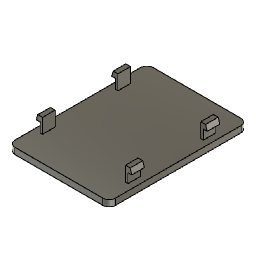
Bottom (Autodesk Fusion 360 design; units mm, degrees)
Autodesk Fusion 360 part; units mm, degrees
sketch "Sketch1" plane through (0, 0, 0) normal (0, 0, 1) x (1, 0, 0)
  line L0 (0, 0) -> (80, 0)
  line L1 (80, 0) -> (80, 110)
  line L2 (80, 110) -> (0, 110)
  line L3 (0, 110) -> (0, 0)
  dimension "d1" = 80
  dimension "d2" = 110
  constraint horizontal L0
  constraint vertical L1
  constraint horizontal L2
  constraint vertical L3
  constraint coincident L0.start L3.end
  measures "d1" distance of L0.start L0.end
  measures "d2" distance of L0.start L2.end
extrude "Extrude1" add sketch "Sketch1" along normal blind 5
fillet "Fillet1" radius 5 4 edges at (80, 0, 2.5) (0, 0, 2.5) (80, 110, 2.5) (0, 110, 2.5)
sketch "Sketch2" plane through (0, 0, 5) normal (0, 0, 1) x (-1, 0, 0)
  arc A0 (-5, -110) -> (0, -105) centre (-5, -105) ccw
  line L0 (0, -105) -> (0, -5)
  arc A1 (0, -5) -> (-5, 0) centre (-5, -5) ccw
  line L1 (-5, 0) -> (-75, 0)
  arc A2 (-75, 0) -> (-80, -5) centre (-75, -5) ccw
  line L2 (-80, -5) -> (-80, -105)
  arc A3 (-80, -105) -> (-75, -110) centre (-75, -105) ccw
  line L3 (-75, -110) -> (-5, -110)
  line L4 (-5, -30) -> (-8, -30)
  line L5 (-8, -30) -> (-8, -20)
  line L6 (-8, -20) -> (-5, -20)
  line L7 (-5, -20) -> (-5, -30)
  line L8 (-5, -90) -> (-8, -90)
  line L9 (-8, -90) -> (-8, -80)
  line L10 (-8, -80) -> (-5, -80)
  line L11 (-5, -80) -> (-5, -90)
  line L12 (0, 0) -> (-40, 0)
  line L13 (-40, 0) -> (-40, -110)
  line L14 (-75, -90) -> (-72, -90)
  line L15 (-72, -90) -> (-72, -80)
  line L16 (-75, -80) -> (-75, -90)
  line L17 (-72, -80) -> (-75, -80)
  line L18 (-75, -30) -> (-72, -30)
  line L19 (-72, -20) -> (-75, -20)
  line L20 (-75, -20) -> (-75, -30)
  line L21 (-72, -30) -> (-72, -20)
  dimension "d7" = 3
  dimension "d8" = 10
  dimension "d9" = 3
  dimension "d10" = 10
  dimension "d11" = 5
  dimension "d12" = 5
  dimension "d13" = 20
  dimension "d14" = 20
  dimension "d15" = 40
  constraint horizontal L4
  constraint vertical L5
  constraint horizontal L6
  constraint vertical L7
  constraint horizontal L8
  constraint vertical L9
  constraint horizontal L10
  constraint vertical L11
  constraint coincident L12.start origin
  constraint parallel L1 L12
  constraint perpendicular L1 L13
  constraint symmetric L4.start L13 L18.start
  constraint symmetric L4.end L13 L18.end
  constraint symmetric L5.end L13 L19.start
  constraint symmetric L6.end L13 L19.end
  constraint symmetric L8.start L13 L14.start
  constraint symmetric L8.end L13 L14.end
  constraint symmetric L9.end L13 L15.end
  constraint symmetric L10.end L13 L16.start
  measures "d7" distance of L4.start L4.end
  measures "d8" distance of L4.start L6.end
  measures "d9" distance of L8.start L8.end
  measures "d10" distance of L8.start L10.end
  measures "d11" distance of L0 L11
  measures "d12" distance of L0 L7
  measures "d13" distance of L1 L6
  measures "d14" distance of L3 L8
  measures "d15" distance of L12.start L12.end
extrude "Extrude2" add sketch "Sketch2" along normal blind 7.5 contours L4 L5 L6 L7 | L8 L9 L10 L11 | L14 L15 L16 L17 | L18 L19 L20 L21
sketch "Sketch3" plane through (0, 20, 0) normal (0, -1, 0) x (1, 0, 0)
  line L0 (5, 5) -> (8, 5)
  line L1 (8, 5) -> (8, 12.5)
  line L2 (8, 12.5) -> (5, 12.5)
  line L3 (5, 12.5) -> (5, 5)
  line L4 (5, 12.5) -> (2, 12.5)
  line L5 (8, 12.5) -> (8, 17.5)
  line L6 (8, 17.5) -> (2, 12.5)
  line L7 (72, 12.5) -> (72, 17.5)
  line L8 (75, 12.5) -> (78, 12.5)
  line L9 (72, 17.5) -> (78, 12.5)
  line L10 (72, 12.5) -> (75, 12.5)
  dimension "d18" = 5
  dimension "d48" = 3
  dimension "d54" = 5
  dimension "d55" = 3
  constraint coincident L2.end L3.start
  constraint perpendicular L3 L4
  constraint coincident L1.end L2.start
  constraint perpendicular L2 L5
  constraint vertical L7
  constraint perpendicular L7 L8
  constraint perpendicular L7 L10
  measures "d18" distance of L1.end L5.end
  measures "d48" distance of L3 L4.end
  measures "d54" distance of L7.start L7.end
  measures "d55" distance of L8.start L8.end
extrude "Extrude3" add sketch "Sketch3" against normal blind 10 contours L2 L4 L5 L6 | L7 L8 L9 L10
sketch "Sketch4" plane through (0, 90, 0) normal (0, 1, 0) x (-1, 0, 0)
  line L0 (-75, 5) -> (-72, 5)
  line L1 (-72, 5) -> (-72, 12.5)
  line L2 (-72, 12.5) -> (-75, 12.5)
  line L3 (-75, 12.5) -> (-75, 5)
  line L4 (-78, 12.5) -> (-72, 17.5)
  line L5 (-72, 17.5) -> (-72, 12.5)
  line L6 (-78, 12.5) -> (-75, 12.5)
  line L7 (-8, 12.5) -> (-5, 12.5)
  line L8 (-5, 12.5) -> (-2, 12.5)
  line L9 (-8, 12.5) -> (-8, 17.5)
  line L10 (-8, 17.5) -> (-2, 12.5)
  dimension "d42" = 5
  dimension "d43" = 3
  dimension "d46" = 3
  dimension "d47" = 3
  dimension "d52" = 5
  constraint coincident L1.end L2.start
  constraint collinear L1 L5
  constraint coincident L2.end L3.start
  constraint perpendicular L3 L6
  constraint parallel L7 L8
  constraint perpendicular L7 L9
  measures "d42" distance of L1.end L4.end
  measures "d43" distance of L4.start L2.end
  measures "d46" distance of L7.start L7.end
  measures "d47" distance of L8.end L7.end
  measures "d52" distance of L7.start L9.end
extrude "Extrude4" add sketch "Sketch4" against normal blind 10 contours L2 L4 L5 L6 | L7 L8 L9 L10
sketch "Sketch9" plane through (0, 90, 0) normal (0, 1, 0) x (-1, 0, 0)
  line L0 (-75, 5) -> (-72, 5)
  line L1 (-72, 5) -> (-72, 17.5)
  line L2 (-72, 17.5) -> (-78, 12.5)
  line L3 (-78, 12.5) -> (-75, 12.5)
  line L4 (-75, 12.5) -> (-75, 5)
  line L5 (-72, 17.5) -> (-76.5, 17.5)
  line L6 (-76.5, 17.5) -> (-78, 12.5)
  line L7 (-72, 17.5) -> (-73, 17.5)
  line L8 (-73, 17.5) -> (-73, 5)
  line L9 (-73, 5) -> (-72, 5)
  line L10 (-72, 5) -> (-72, 17.5)
  line L11 (-73, 16.6667) -> (-76.75, 16.6667)
  dimension "d56" = 4.5
  dimension "d57" = 1
  constraint coincident L1.end L2.start
  constraint perpendicular L1 L5
  constraint coincident L2.end L3.start
  constraint horizontal L7
  constraint vertical L8
  constraint horizontal L9
  constraint vertical L10
  constraint coincident L8 L11.start
  constraint coincident L2 L11.start
  constraint coincident L6 L11.end
  constraint perpendicular L8 L11
  measures "d56" distance of L1.end L5.end
  measures "d57" distance of L1.end L7.end
sketch "Sketch10" plane through (0, 90, 0) normal (0, 1, 0) x (-1, 0, 0)
  line L0 (-8, 5) -> (-5, 5)
  line L1 (-5, 5) -> (-5, 12.5)
  line L2 (-5, 12.5) -> (-2, 12.5)
  line L3 (-2, 12.5) -> (-8, 17.5)
  line L4 (-8, 17.5) -> (-8, 5)
  line L5 (-8, 17.5) -> (-3.5, 17.5)
  line L6 (-3.5, 17.5) -> (-2, 12.5)
  line L7 (-8, 17.5) -> (-7, 17.5)
  line L8 (-7, 17.5) -> (-7, 5)
  line L9 (-7, 5) -> (-8, 5)
  line L10 (-8, 5) -> (-8, 17.5)
  line L11 (-7, 16.6667) -> (-3.25, 16.6667)
  dimension "d58" = 4.5
  dimension "d59" = 1
  constraint coincident L3.end L4.start
  constraint perpendicular L4 L5
  constraint coincident L2.end L3.start
  constraint horizontal L7
  constraint vertical L8
  constraint horizontal L9
  constraint vertical L10
  constraint coincident L3 L11.start
  constraint coincident L8 L11.start
  constraint coincident L6 L11.end
  constraint perpendicular L8 L11
  measures "d58" distance of L3.end L5.end
  measures "d59" distance of L3.end L7.end
extrude "Extrude8" cut sketch "Sketch10" sketch "Sketch9" against normal blind 70 contours L0 L3 L4 L8 L9 L10 | L3 L5 L7 L8 of sketch 2 contours L0 L1 L2 L8 L9 L10 | L2 L5 L7 L8
extrude "Extrude9" add sketch "Sketch10" sketch "Sketch9" against normal blind 70 contours L3 L6 L11 of sketch 2 contours L2 L6 L11
sketch "Sketch11" plane through (0, 0, 0) normal (-1, 0, 0) x (0, -1, 0)
  line L0 (-105, 5) -> (-105, 0)
  line L1 (-105, 0) -> (-5, 0)
  line L2 (-5, 0) -> (-5, 5)
  line L3 (-5, 5) -> (-105, 5)
  line L4 (-110, 5) -> (-80, 5)
  line L5 (-80, 5) -> (-30, 5)
  line L6 (-30, 5) -> (-30, 26)
  line L7 (-30, 26) -> (-80, 26)
  line L8 (-80, 26) -> (-80, 5)
  dimension "d64" = 50
  constraint coincident L3 L4.end
  constraint horizontal L5
  constraint vertical L6
  constraint horizontal L7
  constraint vertical L8
  measures "d64" distance of L4.end L5.end
extrude "Extrude10" cut sketch "Sketch11" against normal blind 100 contours L3 L5 L6 L7 L8
